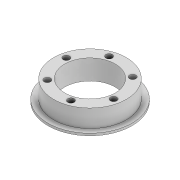
# Autodesk Inventor part: j1FlangeV2
Saved by Autodesk Inventor 2021 (Build 250183000, 183)
## iProperties
Created: 2020-08-08
Part Number: j1FlangeV2
Material: Generic
Document SubType Name: Modeling
Designer: Derm
Density: 1 g/cm^3
Appearance: Default
Mass: 25.0496 g
Surface Area: 120.713 cm^2
Volume: 25.0496 cm^3
Author: Derm
Autodesk Inventor part; units mm, degrees
ref_plane "YZ Plane" through (0, 0, 0) normal (1, 0, 0) x (0, 1, 0)
ref_plane "XZ Plane" through (0, 0, 0) normal (0, 1, 0) x (-1, 0, 0)
ref_plane "XY Plane" through (0, 0, 0) normal (0, 0, 1) x (1, 0, 0)
sketch "Sketch1" plane through (0, 0, 0) normal (0, 1, 0) x (-1, 0, 0)
  circle A0 centre (0, 0) radius 22.5
  circle A1 centre (0, 0) radius 37.5
  dimension "d0" = 45
  dimension "d1" = 75
  constraints: 2 centre point, 2 coincident
  measures "d0" diameter of A0
  measures "d1" diameter of A1
extrude "Extrusion1" add sketch "Sketch1" along normal blind 2
sketch "Sketch2" plane through (0, 2, 0) normal (0, 1, 0) x (1, 0, 0)
  circle A0 centre (0, 0) radius 37.5 projected
  circle A1 centre (0, 0) radius 22.5 projected
  circle A2 centre (0, 0) radius 32.4
  dimension "d4" = 64.8
  constraints: 1 centre point, 1 coincident
  measures "d4" diameter of A2
extrude "Extrusion2" add sketch "Sketch2" along normal blind 15.875 contours A2
feature "FaceDraft1" [suppressed]
sketch "Sketch3" plane through (0, 17.875, 0) normal (0, 1, 0) x (1, 0, 0)
  circle A0 centre (26.4608, -5.3692) radius 2.875 projected
  circle A1 centre (17.8802, 20.2311) radius 2.875 projected
  circle A2 centre (-8.5805, 25.6003) radius 2.875 projected
  circle A3 centre (-26.4608, 5.3692) radius 2.875 projected
  circle A4 centre (-17.8802, -20.2311) radius 2.875 projected
  circle A5 centre (8.5805, -25.6003) radius 2.875 projected
  point P0 (0, 0)
extrude "Extrusion3" cut sketch "Sketch3" against normal through all
sketch "Sketch4" plane through (0, 0, 0) normal (0, -1, 0) x (1, 0, 0)
  circle A0 centre (26.4608, 5.3692) radius 2.875 projected
  line L0 (30.7783, 3.7285) -> (27.1986, 0.8097)
  line L1 (27.1986, 0.8097) -> (22.8811, 2.4504)
  line L2 (22.8811, 2.4504) -> (22.1432, 7.0099)
  line L3 (22.1432, 7.0099) -> (25.7229, 9.9287)
  line L4 (25.7229, 9.9287) -> (30.0404, 8.2879)
  line L5 (30.0404, 8.2879) -> (30.7783, 3.7285)
  point P0 (0, 0)
  dimension "d10" = 8
  constraints: 12 end point, 1 coincident, 13 other
  measures "d10" distance between parallel lines of L1 L4
extrude "Extrusion4" cut sketch "Sketch4" against normal blind 5 contours A0 | L0 L1 L2 L3 L4 L5
pattern_circular "Circular Pattern1" count 6 over 360 about axis through (0, 2, 0) along (0, 1, 0) of "Extrusion4"
body "Solid1"
